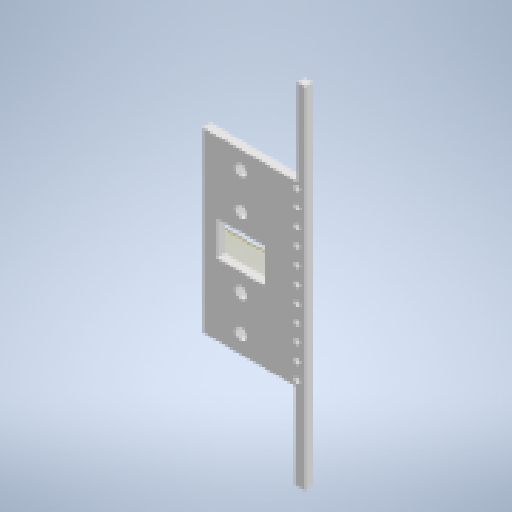
# Autodesk Inventor part: Pièce9
Saved by Autodesk Inventor 2024.2 (Build 282272000, 272)
## iProperties
Created: 2023-12-15
Part Number: Pièce9
Material: Générique
Document SubType Name: Modeling
Designer: eleves
Density: 1 g/cm^3
Appearance: Par défaut
Author: eleves
Autodesk Inventor part; units mm, degrees
ref_plane "YZ Plane" through (0, 0, 0) normal (1, 0, 0) x (0, 1, 0)
ref_plane "XZ Plane" through (0, 0, 0) normal (0, 1, 0) x (-1, 0, 0)
ref_plane "XY Plane" through (0, 0, 0) normal (0, 0, 1) x (1, 0, 0)
ref_plane "Plan de construction1" through (0, 0, 0) normal (0, 0, 1) x (1, 0, 0)
sketch "Esquisse1" plane through (0, 0, 0) normal (0, 0, 1) x (1, 0, 0)
  line L0 (29.95, -1) -> (16.05, -1) projected
  line L1 (23, -1) -> (61.5, -1) construction
  circle A0 centre (23, 10.75) radius 3.5056 projected
  circle A1 centre (23, 32.25) radius 3.5056 projected
  line L2 (0, 0) -> (46, 0) projected
  line L3 (37.5, 43) -> (37.5, 53) projected
  line L4 (8.5, 43) -> (37.5, 43) projected
  line L5 (8.5, 43) -> (8.5, 53) projected
  line L6 (0, 0) -> (0, 53) projected
  circle A2 centre (23, 95.85) radius 3.5056 projected
  circle A3 centre (23, 74.35) radius 3.5056 projected
  line L7 (0, 106.6) -> (46, 106.6) projected
  line L8 (0, 106.6) -> (0, 53.6) projected
  line L9 (8.5, 63.6) -> (8.5, 53.6) projected
  line L10 (8.5, 63.6) -> (37.5, 63.6) projected
  line L11 (37.5, 63.6) -> (37.5, 53.6) projected
  line L12 (8.5, 53.6) -> (8.5, 53)
  line L13 (37.5, 53.6) -> (37.5, 53)
  line L14 (61.5, -51.7) -> (61.5, 158.3)
  line L15 (37.5, 53.3) -> (61.5, 53.3) construction
  line L16 (61.5, 158.3) -> (56.5, 158.3)
  line L17 (56.5, 158.3) -> (56.5, 106.6)
  line L18 (56.5, 106.6) -> (46, 106.6)
  line L19 (55.4096, 0) -> (55.4096, -51.7)
  line L20 (55.4096, -51.7) -> (61.5, -51.7)
  line L21 (55.4096, 0) -> (46, 0)
  circle A4 centre (56.5, 53.3) radius 1.75
  line L22 (37.5, 63.3) -> (61.5, 63.3) construction
  circle A5 centre (56.5, 63.3) radius 1.75
  line L23 (37.5, 73.3) -> (61.5, 73.3) construction
  circle A6 centre (56.5, 73.3) radius 1.75
  line L24 (37.5, 83.3) -> (61.5, 83.3) construction
  circle A7 centre (56.5, 83.3) radius 1.75
  line L25 (37.5, 93.3) -> (61.5, 93.3) construction
  circle A8 centre (56.5, 93.3) radius 1.75
  line L26 (37.5, 103.3) -> (61.5, 103.3) construction
  circle A9 centre (56.5, 103.3) radius 1.75
  line L27 (37.5, 43.3) -> (61.5, 43.3) construction
  circle A10 centre (56.5, 43.3) radius 1.75
  line L28 (37.5, 53.3) -> (61.5, 53.3) construction
  circle A11 centre (56.5, 53.3) radius 1.75
  line L29 (37.5, 63.3) -> (61.5, 63.3) construction
  circle A12 centre (56.5, 63.3) radius 1.75
  line L30 (37.5, 73.3) -> (61.5, 73.3) construction
  circle A13 centre (56.5, 73.3) radius 1.75
  line L31 (37.5, 83.3) -> (61.5, 83.3) construction
  circle A14 centre (56.5, 83.3) radius 1.75
  line L32 (37.5, 93.3) -> (61.5, 93.3) construction
  circle A15 centre (56.5, 93.3) radius 1.75
  line L33 (37.5, 33.3) -> (61.5, 33.3) construction
  circle A16 centre (56.5, 33.3) radius 1.75
  line L34 (37.5, 43.3) -> (61.5, 43.3) construction
  circle A17 centre (56.5, 43.3) radius 1.75
  line L35 (37.5, 53.3) -> (61.5, 53.3) construction
  circle A18 centre (56.5, 53.3) radius 1.75
  line L36 (37.5, 63.3) -> (61.5, 63.3) construction
  circle A19 centre (56.5, 63.3) radius 1.75
  line L37 (37.5, 73.3) -> (61.5, 73.3) construction
  circle A20 centre (56.5, 73.3) radius 1.75
  line L38 (37.5, 83.3) -> (61.5, 83.3) construction
  circle A21 centre (56.5, 83.3) radius 1.75
  line L39 (37.5, 23.3) -> (61.5, 23.3) construction
  circle A22 centre (56.5, 23.3) radius 1.75
  line L40 (37.5, 33.3) -> (61.5, 33.3) construction
  circle A23 centre (56.5, 33.3) radius 1.75
  line L41 (37.5, 43.3) -> (61.5, 43.3) construction
  circle A24 centre (56.5, 43.3) radius 1.75
  line L42 (37.5, 53.3) -> (61.5, 53.3) construction
  circle A25 centre (56.5, 53.3) radius 1.75
  line L43 (37.5, 63.3) -> (61.5, 63.3) construction
  circle A26 centre (56.5, 63.3) radius 1.75
  line L44 (37.5, 73.3) -> (61.5, 73.3) construction
  circle A27 centre (56.5, 73.3) radius 1.75
  line L45 (37.5, 13.3) -> (61.5, 13.3) construction
  circle A28 centre (56.5, 13.3) radius 1.75
  line L46 (37.5, 23.3) -> (61.5, 23.3) construction
  circle A29 centre (56.5, 23.3) radius 1.75
  line L47 (37.5, 33.3) -> (61.5, 33.3) construction
  circle A30 centre (56.5, 33.3) radius 1.75
  line L48 (37.5, 43.3) -> (61.5, 43.3) construction
  circle A31 centre (56.5, 43.3) radius 1.75
  line L49 (37.5, 53.3) -> (61.5, 53.3) construction
  circle A32 centre (56.5, 53.3) radius 1.75
  line L50 (37.5, 63.3) -> (61.5, 63.3) construction
  circle A33 centre (56.5, 63.3) radius 1.75
  line L51 (37.5, 3.3) -> (61.5, 3.3) construction
  circle A34 centre (56.5, 3.3) radius 1.75
  line L52 (37.5, 13.3) -> (61.5, 13.3) construction
  circle A35 centre (56.5, 13.3) radius 1.75
  line L53 (37.5, 23.3) -> (61.5, 23.3) construction
  circle A36 centre (56.5, 23.3) radius 1.75
  line L54 (37.5, 33.3) -> (61.5, 33.3) construction
  circle A37 centre (56.5, 33.3) radius 1.75
  line L55 (37.5, 43.3) -> (61.5, 43.3) construction
  circle A38 centre (56.5, 43.3) radius 1.75
  line L56 (37.5, 53.3) -> (61.5, 53.3) construction
  circle A39 centre (56.5, 53.3) radius 1.75
  line L57 (0, 53) -> (0, 53.6)
  dimension "d0" = 38.5
  dimension "d2" = 210
  dimension "d3" = 105
  dimension "d4" = 5
  dimension "d5" = 5
  dimension "d6" = 3.5
  dimension "d9" = 10
  dimension "d12" = 10
  constraints: 94 end point, 36 centre point, 36 point on line, 7 vertical, 3 midpoint, 3 perpendicular, 2 horizontal, 2 parallel, 175 other
  measures "d0" distance of L1.start L1.end
  measures "d2" distance of L14.start L14.end
  measures "d3" distance from line of L14.start L15
  measures "d4" distance of L14.end L16.end
  measures "d5" distance from line of L14 A4.centre
  measures "d6" diameter of A4
  measures "d9" distance of L15.start L22.start
  measures "d12" distance of L15.start L27.start
extrude "Extrusion1" add sketch "Esquisse1" along normal blind 5
